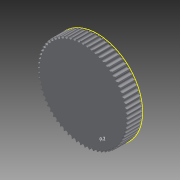
# Autodesk Inventor part: HTD3-66T stock a_6a22m066tm20
Saved by Autodesk Inventor 2015 (Build 190159000, 159)
## iProperties
Created: 2015-04-17
Part Number: HTD3-66T stock a_6a22m066tm20
Material: Generic
Document SubType Name: Modeling
Designer: doctor
Density: 1 g/cm^3
Appearance: Default
Author: carefree
Title: A_6A22M066TM20
Sending System: PRO/ENGINEER BY PARAMETRIC TECHNOLOGY CORPORATION, 2010020
Preprocessor: PRO/ENGINEER BY PARAMETRIC TECHNOLOGY CORPORATION, 2010020
Thickness: 10.000 mm
Author: doctor
Autodesk Inventor part; units mm, degrees
ref_plane "YZ Plane" through (0, 0, 0) normal (1, 0, 0) x (0, 1, 0)
ref_plane "XZ Plane" through (0, 0, 0) normal (0, 1, 0) x (-1, 0, 0)
ref_plane "XY Plane" through (0, 0, 0) normal (0, 0, 1) x (1, 0, 0)
sketch "Projected66TProfile" plane through (0, 0, 0) normal (0, 0, 1) x (1, 0, 0)
  arc A0 (6.7103, -30.0564) -> (7.1441, -30.3248) centre (7.0614, -29.9738) ccw projected
  arc A1 (7.1441, -30.3248) -> (1.6888, -31.1092) centre (0, 0) ccw projected
  arc A2 (1.6888, -31.1092) -> (2.0294, -30.7294) centre (1.6692, -30.749) ccw projected
  arc A3 (2.8337, -29.6757) -> (2.0294, -30.7294) centre (3.0489, -30.6739) ccw projected
  arc A4 (3.8229, -30.5582) -> (2.8337, -29.6757) centre (2.8112, -30.6966) ccw projected
  arc A5 (3.8229, -30.5582) -> (4.2292, -30.8666) centre (4.1803, -30.5093) ccw projected
  arc A6 (4.2292, -30.8666) -> (4.6382, -30.8078) centre (0, 0) ccw projected
  arc A7 (4.6382, -30.8078) -> (4.9412, -30.3974) centre (4.5845, -30.4511) ccw projected
  arc A8 (5.6417, -29.272) -> (4.9412, -30.3974) centre (5.9509, -30.2452) ccw projected
  arc A9 (6.7103, -30.0564) -> (5.6417, -29.272) centre (5.7164, -30.2903) ccw projected
  circle A10 centre (0, 0) radius 9.55 projected
  circle A11 centre (0, 0) radius 31.155
  constraints: 1 centre point, 1 coincident, 1 concentric
sketch "ProfileModifiedForPrinter" plane through (0, 0, 0) normal (0, 0, 1) x (1, 0, 0)
  arc A0 (1.6888, -31.1092) -> (2.0294, -30.7294) centre (1.6692, -30.749) ccw construction
  arc A1 (2.8337, -29.6757) -> (2.0294, -30.7294) centre (3.0489, -30.6739) ccw construction
  arc A2 (3.8229, -30.5582) -> (2.8337, -29.6757) centre (2.8112, -30.6966) ccw construction
  arc A3 (3.8229, -30.5582) -> (4.2292, -30.8666) centre (4.1803, -30.5093) ccw construction
  arc A4 (4.2292, -30.8666) -> (4.6382, -30.8078) centre (0, 0) ccw construction
  circle A5 centre (0, 0) radius 31.155 projected
  arc A6 (2.8146, -29.4755) -> (1.8297, -30.7403) centre (3.0489, -30.6739) ccw
  arc A7 (4.0211, -30.5311) -> (2.8146, -29.4755) centre (2.8112, -30.6966) ccw
  arc A8 (1.4874, -31.1195) -> (1.8297, -30.7403) centre (1.4702, -30.7599) ccw
  line L0 (1.4702, -30.7599) -> (1.8297, -30.7403) construction
  arc A9 (4.0211, -30.5311) -> (4.4289, -30.8386) centre (4.3777, -30.4823) ccw
  line L1 (4.3777, -30.4823) -> (4.0211, -30.5311) construction
  dimension "PrinterOverextrusionCorrection" = 0.2
  constraints: 10 point on circle, 4 centre point, 4 end point, 4 tangent, 2 point on line, 1 other
  measures "PrinterOverextrusionCorrection" radial gap between concentric circles of A2 A7
extrude "Base" add sketch "ProfileModifiedForPrinter" along normal blind 10
extrude "Extrusion4" cut sketch "ProfileModifiedForPrinter" along normal through all contours A8 A6 A7 A9 A5 picked at (3.0085, -30.5103)
pattern_circular "Circular Pattern2" count 66 over 360 about axis through (0, 0, -10) along (0, 0, 1) of "Extrusion4"
body "Solid1"
